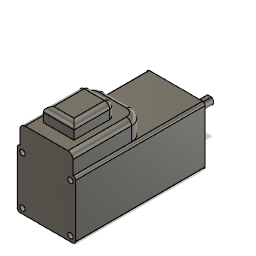
Mouting Plate BOB 2 v3 (35cm long max.) (Autodesk Fusion 360 archive; units mm, degrees)
design "NEMA 23 Integrated Easy Servo Motor 130w"
Autodesk Fusion 360 part; units mm, degrees
sketch "Sketch1" plane through (0, 0, 0) normal (0, 0, 1) x (1, 0, 0)
  line L0 (0, 0) -> (57.15, 0)
  line L1 (57.15, 0) -> (57.15, 57.15)
  line L2 (57.15, 57.15) -> (0, 57.15)
  line L3 (0, 57.15) -> (0, 0)
  circle A0 centre (52.125, 52.125) radius 2.6
  line L4 (28.575, 0) -> (28.575, 57.15) construction
  line L5 (0, 28.575) -> (57.15, 28.575) construction
  circle A1 centre (5.025, 52.125) radius 2.6
  circle A2 centre (5.025, 5.025) radius 2.6
  circle A3 centre (52.125, 5.025) radius 2.6
  circle A4 centre (28.575, 28.575) radius 19.05
  line L6 (2.575, 57.15) -> (54.575, 57.15)
  line L7 (54.575, 57.15) -> (54.575, 76)
  line L8 (54.575, 76) -> (2.575, 76)
  line L9 (2.575, 76) -> (2.575, 57.15)
  circle A5 centre (28.575, 28.575) radius 4
  line L10 (26.6385, 32.075) -> (30.5115, 32.075)
  line L11 (13.575, 76) -> (43.575, 76)
  line L12 (43.575, 76) -> (43.575, 89.67)
  line L13 (43.575, 89.67) -> (13.575, 89.67)
  line L14 (13.575, 89.67) -> (13.575, 76)
  point P0 (47.5479, 45.3005)
  dimension "d1" = 57.15
  dimension "d2" = 57.15
  dimension "d3" = 5.2
  dimension "d5" = 5.2
  dimension "d6" = 47.1
  dimension "d8" = 5.2
  dimension "d10" = 47.1
  dimension "d12" = 5.2
  dimension "d13" = 47.1
  dimension "d14" = 47.1
  dimension "d15" = 38.1
  dimension "d16" = 76
  dimension "d17" = 8
  dimension "d19" = 3.5
  dimension "d20" = 52
  dimension "d21" = 13.67
  dimension "d22" = 30
  constraint horizontal L0
  constraint vertical L1
  constraint horizontal L2
  constraint vertical L3
  constraint coincident L0.start L3.end
  constraint midpoint L0 L4.start
  constraint midpoint L2 L4.end
  constraint midpoint L3 L5.start
  constraint midpoint L1 L5.end
  constraint symmetric A0 L4 A1
  constraint symmetric L5 A1.centre A2.centre
  constraint midpoint L5 A4.centre
  constraint horizontal L6
  constraint vertical L7
  constraint horizontal L8
  constraint vertical L9
  constraint coincident L2 L6.start
  constraint concentric A4 A5
  constraint coincident A5 L10.start
  constraint coincident A5 L10.end
  constraint perpendicular L4 L10
  constraint symmetric L4 L7 L9
  constraint horizontal L11
  constraint vertical L12
  constraint horizontal L13
  constraint vertical L14
  constraint coincident L8 L11.start
  constraint symmetric L4 L12 L14
  measures "d1" distance of L0.start L0.end
  measures "d2" distance of L0.start L2.end
  measures "d3" diameter of A0
  measures "d5" diameter of A1
  measures "d6" distance of A0.centre A1.centre
  measures "d8" diameter of A2
  measures "d10" distance of A1.centre A2.centre
  measures "d12" diameter of A3
  measures "d13" horizontal distance of A2.centre A3.centre
  measures "d14" distance of A0.centre A3.centre
  measures "d15" diameter of A4
  measures "d16" distance of L0 L8
  measures "d17" diameter of A5
  measures "d19" distance of L5 L10
  measures "d20" distance of L7.end L8.end
  measures "d21" distance of L11.start L13.end
  measures "d22" distance of L12.end L13.end
extrude "Extrude1" add sketch "Sketch1" along normal blind 127 contours L0 L1 L2 L3 L6 | A4 | A5 L10 | A5 L10
fillet "Fillet1" radius 2.5 4 edges at (57.15, 57.15, 63.5) (57.15, 0, 63.5) (0, 0, 63.5) (0, 57.15, 63.5)
extrude "Extrude2" add sketch "Sketch1" against normal blind 70 from surface at 127 contours L2 L6 L7 L8 L9 L11
fillet "Fillet2" radius 12.5 2 edges at (54.575, 66.575, 57) (2.575, 66.575, 57)
fillet "Fillet2" radius 5 3 edges at (54.575, 76, 92) (28.575, 76, 57) (2.575, 76, 92)
extrude "Extrude3" add sketch "Sketch1" along normal blind 40 from surface at 75 contours L8 L11 L12 L13 L14
fillet "Fillet3" radius 5 6 edges at (43.575, 89.67, 95) (43.575, 82.835, 75) (13.575, 82.835, 75) (28.575, 89.67, 75) (13.575, 89.67, 95) (28.575, 89.67, 115)
extrude "Extrude4" add sketch "Sketch1" against normal blind 2 contours A4 | A5 L10 | A5 L10
extrude "Extrude5" add sketch "Sketch1" against normal blind 33 contours A5 L10 picked at (29.5161, 29.5962)
extrude "Extrude6" add sketch "Sketch1" against normal blind 6 contours A5 L10 picked at (28.1041, 32.1557)
equation "d10 = d6"
equation "d12 = d3"
equation "d13 = d6"
equation "d14 = d6"
equation "d19 = 7.5 mm - ( d17 / 2 )"
equation "d44 = ( -1 * ( 33 - 27 ) ) * 1 mm"

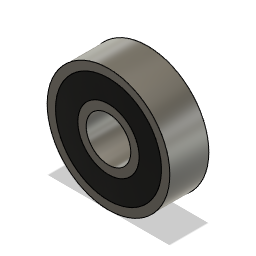
design "608 Bearings"
Autodesk Fusion 360 part; units mm, degrees
sketch "Sketch1" plane through (0, 0, 0) normal (0, 0, 1) x (1, 0, 0)
  circle A0 centre (0, 0) radius 11
  circle A1 centre (0, 0) radius 9.5
  circle A2 centre (0, 0) radius 4
  circle A3 centre (0, 0) radius 5.5
  dimension "d1" = 22
  dimension "d2" = -1.5
  dimension "d3" = 8
  dimension "d4" = 1.5
  constraint coincident A0.centre A1.centre
  measures "d1" diameter of A0
  measures "d3" diameter of A2
extrude "Extrude1" add sketch "Sketch1" along normal blind 7 makes body 1 at (5.4727, -0.5476, 4.6667) makes body 2 at (10.9453, -1.0952, 4.6667)
extrude "Extrude2" add sketch "Sketch1" along normal blind 7 separate body contours A1 makes body 3

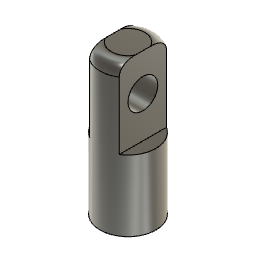
design "I-Joit"
Autodesk Fusion 360 part; units mm, degrees
sketch "Boceto1" plane through (0, 0, 0) normal (0, 0, 1) x (1, 0, 0)
  circle A0 centre (0, 0) radius 7.5
  circle A1 centre (0, 0) radius 4
  dimension "d58" = 15
  dimension "d59" = 8
  constraint coincident A0.centre A1.centre
  constraint concentric A0 A1
  measures "d58" diameter of A0
  measures "d59" diameter of A1
extrude "Extruir12" add sketch "Boceto1" along normal blind 40 contours A0 | A1
extrude "Extruir13" cut sketch "Boceto1" along normal blind 15 contours A1
sketch "Boceto16" plane through (0, 0, 40) normal (0, 0, 1) x (-1, 0, 0)
  circle A0 centre (0, 0) radius 7.5
  line L0 (-4, -12.0799) -> (4, -12.0799)
  line L1 (4, -12.0799) -> (4, 12.0799)
  line L2 (4, 12.0799) -> (-4, 12.0799)
  line L3 (-4, 12.0799) -> (-4, -12.0799)
  line L4 (-4, -12.0799) -> (4, 12.0799) construction
  line L5 (4, -12.0799) -> (-4, 12.0799) construction
  line L6 (-8.5026, -18.8703) -> (8.5026, -18.8703)
  line L7 (8.5026, -18.8703) -> (8.5026, 18.8703)
  line L8 (8.5026, 18.8703) -> (-8.5026, 18.8703)
  line L9 (-8.5026, 18.8703) -> (-8.5026, -18.8703)
  line L10 (-8.5026, -18.8703) -> (8.5026, 18.8703) construction
  line L11 (8.5026, -18.8703) -> (-8.5026, 18.8703) construction
  dimension "d64" = 8
  constraint horizontal L0
  constraint perpendicular L0 L1
  constraint parallel L0 L2
  constraint parallel L1 L3
  constraint coincident L4 A0.centre
  constraint coincident L5 A0.centre
  constraint coincident A0.centre origin
  constraint horizontal L6
  constraint perpendicular L6 L7
  constraint parallel L6 L8
  constraint parallel L7 L9
  constraint coincident L10 A0.centre
  constraint coincident L11 A0.centre
  measures "d64" distance of L1.end L2.end
extrude "Extruir14" cut sketch "Boceto16" against normal blind 21 contours A0 L1 | A0 L3 | L6 L7 L8 L9
sketch "Boceto17" plane through (-4, 0, 0) normal (-1, 0, 0) x (0, -1, 0)
  line L0 (-6.3443, 40) -> (-6.3443, 19)
  line L1 (-6.3443, 19) -> (6.3443, 19)
  line L2 (6.3443, 19) -> (6.3443, 40)
  line L3 (6.3443, 40) -> (-6.3443, 40)
  circle A0 centre (0, 30) radius 4
  line L4 (7.5, 0) -> (-7.5, 0)
  dimension "d67" = 8
  dimension "d68" = 30
  measures "d67" diameter of A0
  measures "d68" distance of A0.centre L4
extrude "Extruir15" cut sketch "Boceto17" against normal blind 10 contours A0
fillet "Empalme4" radius 3 2 edges at (0, -7.5, 40) (0, 7.5, 40)

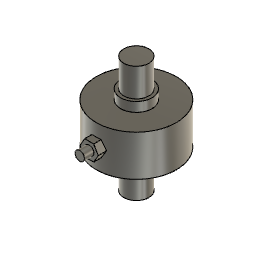
design "Load Cell Mini (200 kg)"
Autodesk Fusion 360 part; units mm, degrees
sketch "Boceto1" plane through (0, 0, 0) normal (0, 0, 1) x (1, 0, 0)
  circle A0 centre (0, 0) radius 12.7
  dimension "d1" = 25.4
  constraint coincident A0.centre origin
  measures "d1" diameter of A0
extrude "Extruir1" add sketch "Boceto1" along normal blind 13
sketch "Boceto2" plane through (0, 0, 13) normal (0, 0, 1) x (-1, 0, 0)
  circle A0 centre (0, 0) radius 12.7
  circle A1 centre (0, 0) radius 5
  dimension "d4" = 10
  constraint coincident A0.centre A1.centre
  measures "d4" diameter of A1
extrude "Extruir2" add sketch "Boceto2" along normal blind 3 contours A1
sketch "Boceto3" plane through (0, 0, 16) normal (0, 0, 1) x (-1, 0, 0)
  circle A0 centre (0, 0) radius 5
  circle A1 centre (0, 0) radius 4
  dimension "d7" = 8
  constraint coincident A0.centre A1.centre
  measures "d7" diameter of A1
extrude "Extruir3" add sketch "Boceto3" along normal blind 9 contours A1
sketch "Boceto4" plane through (0, 0, 0) normal (0, 0, -1) x (1, 0, 0)
  circle A0 centre (0, 0) radius 12.7
  circle A1 centre (0, 0) radius 4
  dimension "d10" = 8
  constraint coincident A0.centre A1.centre
  measures "d10" diameter of A1
extrude "Extruir4" add sketch "Boceto4" along normal blind 12 contours A1
sketch "Boceto5" plane through (0, 0, 0) normal (0, 1, 0) x (1, 0, 0)
  line L0 (-1.4434, -4) -> (-2.8868, -6.5)
  line L1 (-2.8868, -6.5) -> (-1.4434, -9)
  line L2 (-1.4434, -9) -> (1.4434, -9)
  line L3 (1.4434, -9) -> (2.8868, -6.5)
  line L4 (2.8868, -6.5) -> (1.4434, -4)
  line L5 (1.4434, -4) -> (-1.4434, -4)
  line L6 (-12.7, 0) -> (12.7, 0)
  point P0 (0, -6.5)
  dimension "d15" = 6.5
  dimension "d16" = 5
  measures "d15" distance of P0 L6
  measures "d16" distance of L2 L5
extrude "Extruir5" add sketch "Boceto5" against normal blind 15
sketch "Boceto6" plane through (0, -15, 0) normal (0, -1, 0) x (1, 0, 0)
  line L0 (-1.4434, 4) -> (1.4434, 4)
  line L1 (1.4434, 4) -> (2.8868, 6.5)
  line L2 (2.8868, 6.5) -> (1.4434, 9)
  line L3 (1.4434, 9) -> (-1.4434, 9)
  line L4 (-1.4434, 9) -> (-2.8868, 6.5)
  line L5 (-2.8868, 6.5) -> (-1.4434, 4)
  circle A0 centre (0, 6.5) radius 1.5
  dimension "d17" = 3
  measures "d17" diameter of A0
extrude "Extruir6" add sketch "Boceto6" along normal blind 3 contours A0

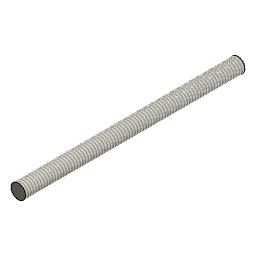
design "8mm T8 Lead Screw (120mm) v1"
Autodesk Fusion 360 part; units mm, degrees
sketch "Sketch1" plane through (0, 0, 0) normal (0, 0, 1) x (1, 0, 0)
  circle A0 centre (0, 0) radius 4
  dimension "d1" = 8
  constraint coincident A0.centre origin
  measures "d1" diameter of A0
extrude "Extrude1" add sketch "Sketch1" along normal blind 120
thread "Thread1" "ISO Metric Trapezoidal Threads 8.0 TR8x1.5 7e" major diameter 7.925 minor diameter 6.0605 pitch 1.5 angle 30 resizes the face on face at (3.9801, -0.3983, 80)

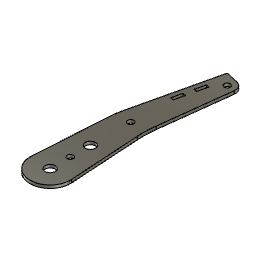
design "Pedal Inox 2"
Autodesk Fusion 360 part; units mm, degrees
sketch "Boceto1" plane through (0, 0, 0) normal (0, 0, 1) x (1, 0, 0)
  circle A0 centre (40.124, 0.0001) radius 5
  circle A1 centre (40.124, 20) radius 3
  circle A2 centre (40.124, 80) radius 3
  arc A3 (20.1636, 1.2575) -> (60.0845, 1.2575) centre (40.124, 0.0001) ccw
  circle A4 centre (40.124, 40) radius 5
  line L0 (45.7789, 149.5191) -> (48.7988, 148.8188)
  line L1 (48.7988, 148.8188) -> (46.5173, 138.9799)
  line L2 (46.5173, 138.9799) -> (43.4975, 139.6801)
  line L3 (43.4975, 139.6801) -> (45.7789, 149.5191)
  line L4 (42.1351, 120.0813) -> (39.1152, 120.7816)
  line L5 (44.4166, 129.9203) -> (42.1351, 120.0813)
  line L6 (39.1152, 120.7816) -> (41.3967, 130.6205)
  line L7 (41.3967, 130.6205) -> (44.4166, 129.9203)
  circle A5 centre (56.6452, 159.3178) radius 3
  line L8 (0, 0) -> (99.8118, 0) construction
  line L9 (40.124, 0.0001) -> (40.124, 227.9121) construction
  line L10 (45.9935, 170) -> (65.9935, 170) construction
  line L11 (40.124, 80) -> (61.8301, 203.101) construction
  line L12 (25.124, 80) -> (55.124, 80) construction
  line L13 (25.124, 80) -> (20.1636, 1.2575)
  line L14 (55.124, 80) -> (60.0845, 1.2575)
  line L15 (25.124, 80) -> (45.9935, 170)
  line L16 (55.124, 80) -> (65.4486, 165.4887)
  line L17 (45.9935, 170) -> (65.4486, 165.4887)
  point P0 (45.9935, 170)
  point P1 (55.9935, 170)
  dimension "d7" = 6
  dimension "d20" = 60
  dimension "d22" = 20
  dimension "d23" = 10
  dimension "d37" = 3.1
  dimension "d39" = 10.1
  dimension "d55" = 40
  dimension "d58" = 20
  dimension "d60" = 170
  dimension "d61" = 20
  dimension "d62" = 9.3
  dimension "d84" = 125
  dimension "d85" = 30
  dimension "d86" = 80
  dimension "d87" = 100
  dimension "d89" = 3.1
  dimension "d90" = 10.1
  dimension "d91" = 20
  dimension "d100" = 8
  dimension "d101" = 8
  constraint coincident P0 L10.start
  constraint equal A1 A2
  constraint concentric A0 A3
  constraint equal A0 A4
  constraint coincident L8.start origin
  constraint vertical L9
  constraint coincident A0.centre A3.centre
  constraint perpendicular L9 L10
  constraint midpoint L10 P1
  constraint coincident A4.centre L9
  constraint coincident A1.centre L9
  constraint coincident A2.centre L9
  constraint perpendicular L0 L3
  constraint perpendicular L0 L1
  constraint perpendicular L1 L2
  constraint coincident A2.centre L11.start
  constraint horizontal L12
  constraint tangent A3 L13
  constraint tangent A3 L14
  constraint coincident P1 L11
  constraint parallel L3 L5
  constraint parallel L3 L15
  constraint collinear L3 L6
  constraint perpendicular L15 L17
  measures "d7" diameter of A1
  measures "d20" distance of A1.centre A2.centre
  measures "d22" radius of A3
  measures "d23" diameter of A0
  measures "d37" distance of L0.start L0.end
  measures "d39" distance of L0.start L2.end
  measures "d55" distance of A4.centre L8
  measures "d58" distance of P0 L10.end
  measures "d60" distance of L8 P1
  measures "d61" distance of A1.centre L8
  measures "d62" distance of L2 L7
  measures "d84" distance of A2.centre L11.end
  measures "d85" distance of L12.start L12.end
  measures "d86" distance of L8 L12
  measures "d87" angle of L8 L11
  measures "d89" distance of L4.start L4.end
  measures "d90" distance of L4.end L6.end
  measures "d91" distance of L0 P0
  measures "d100" distance of A5.centre L17
  measures "d101" distance of A5.centre L16
extrude "Extruir1" add sketch "Boceto1" along normal blind 3
fillet "Empalme2" radius 100 2 edges at (25.124, 80, 1.5) (55.124, 80, 1.5)
fillet "Empalme2" radius 8 1 edges at (65.4486, 165.4887, 1.5)

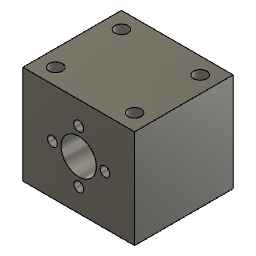
design "Lead Screw Nut Mount"
Autodesk Fusion 360 part; units mm, degrees
sketch "Sketch1" plane through (0, 0, 0) normal (0, 0, 1) x (1, 0, 0)
  circle A0 centre (0, 4) radius 5.375
  line L0 (-17, -11) -> (17, -11)
  line L1 (17, -11) -> (17, 19)
  line L2 (17, 19) -> (-17, 19)
  line L3 (-17, 19) -> (-17, -11)
  circle A1 centre (0, 12) radius 1.5
  circle A2 centre (-8, 4) radius 1.5
  circle A3 centre (0, -4) radius 1.5
  circle A4 centre (8, 4) radius 1.5
  dimension "d5" = 10.75
  dimension "d9" = 3
  dimension "d27" = 34
  dimension "d37" = 30
  constraint horizontal L0
  constraint vertical L1
  constraint horizontal L2
  constraint vertical L3
  measures "d5" diameter of A0
  measures "d9" diameter of A1
  measures "d27" distance of L1 L3
  measures "d37" distance of L0.end L1.end
extrude "Extrude1" add sketch "Sketch1" along normal blind 30
sketch "Sketch2" plane through (17, 0, 0) normal (1, 0, 0) x (0, 0, -1)
  line L0 (0, -11) -> (0, 19)
  line L1 (0, 19) -> (-30, 19)
  line L2 (-30, 19) -> (-30, -11)
  line L3 (-30, -11) -> (0, -11)
  circle A0 centre (-15, 44) radius 5
  line L4 (-15, 19) -> (-15, 44) construction
  circle A1 centre (-15, 44) radius 12.5
  line L5 (-30, 19) -> (-27.4409, 45.2145)
  line L6 (0, 19) -> (-2.5591, 45.2145)
  dimension "d20" = 10
  dimension "d35" = 25
  dimension "d36" = 25
  constraint midpoint L1 L4.start
  constraint perpendicular L1 L4
  constraint coincident A0.centre L4.end
  constraint concentric A0 A1
  constraint coincident L1.end L2.start
  constraint coincident A1 L5.end
  constraint tangent A1 L5
  constraint coincident L0.end L1.start
  constraint coincident A1 L6.end
  constraint tangent A1 L6
  measures "d20" diameter of A0
  measures "d35" distance of L4.start A0.centre
  measures "d36" diameter of A1
sketch "Boceto4" plane through (0, 19, 0) normal (0, 1, 0) x (-1, 0, 0)
  line L0 (-17, 0) -> (17, 0)
  line L1 (17, 0) -> (17, 30)
  line L2 (17, 30) -> (-17, 30)
  line L3 (-17, 30) -> (-17, 0)
  line L4 (-12, 25) -> (12, 25) construction
  line L5 (12, 25) -> (12, 5) construction
  line L6 (12, 5) -> (-12, 5) construction
  line L7 (-12, 5) -> (-12, 25) construction
  circle A0 centre (-12, 25) radius 2
  circle A1 centre (12, 25) radius 2
  circle A2 centre (12, 5) radius 2
  circle A3 centre (-12, 5) radius 2
  dimension "d40" = 24
  dimension "d41" = 20
  dimension "d42" = 5
  dimension "d43" = 5
  dimension "d44" = 4
  constraint horizontal L4
  constraint vertical L5
  constraint horizontal L6
  constraint vertical L7
  constraint coincident L4.start L7.end
  constraint coincident L4.end L5.start
  constraint coincident L5.end L6.start
  constraint coincident L6.end L7.start
  constraint equal A0 A3
  constraint equal A1 A3
  constraint equal A2 A3
  measures "d40" distance of L4.start L4.end
  measures "d41" distance of L4.end L5.end
  measures "d42" distance of L3 L7
  measures "d43" distance of L0 L6
  measures "d44" diameter of A3
extrude "Extruir4" cut sketch "Boceto4" against normal blind 4 contours A0 | A1 | A2 | A3
equation "Screw_Nut_Dia = 10 mm"
equation "Screw_Nut_bolt_Dia = 3 mm"
equation "Screw_Nut_Bolt_Pattern = 16 mm"
equation "d5 = Screw_Nut_Dia + 0.75 mm"
equation "d9 = Screw_Nut_bolt_Dia"
equation "d13 = Screw_Nut_bolt_Dia"
